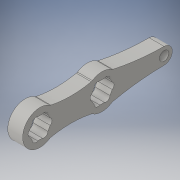
# Autodesk Inventor part: Kevin_CAD_test
Saved by Autodesk Inventor 2016 (Build 200138000, 138)
## iProperties
Created: 2018-06-19
Part Number: Kevin_CAD_test
Material: Generic
Document SubType Name: Modeling
Designer: Student
Density: 1 g/cm^3
Appearance: Default
Author: Student
Autodesk Inventor part; units mm, degrees
ref_plane "YZ Plane" through (0, 0, 0) normal (1, 0, 0) x (0, 1, 0)
ref_plane "XZ Plane" through (0, 0, 0) normal (0, 1, 0) x (-1, 0, 0)
ref_plane "XY Plane" through (0, 0, 0) normal (0, 0, 1) x (1, 0, 0)
sketch "Sketch1" plane through (0, 0, 0) normal (1, 0, 0) x (0, 1, 0)
  arc A0 (14.7437, -9.9374) -> (-14.7437, -9.9374) centre (0, 0) ccw
  arc A1 (-8.382, -127) -> (8.382, -127) centre (0, -127) ccw
  line L0 (-3.2996, -10.4245) -> (-7.3781, -8.0697)
  line L1 (-10.6776, -2.3547) -> (-10.6776, 2.3547)
  line L2 (-7.3781, 8.0697) -> (-3.2996, 10.4245)
  line L3 (3.2996, 10.4245) -> (7.3781, 8.0697)
  line L4 (10.6776, 2.3547) -> (10.6776, -2.3547)
  line L5 (7.3781, -8.0697) -> (3.2996, -10.4245)
  arc A2 (10.6776, 2.3547) -> (7.3781, 8.0697) centre (7.3781, 4.2597) ccw
  arc A3 (7.3781, -8.0697) -> (10.6776, -2.3547) centre (7.3781, -4.2597) ccw
  arc A4 (3.2996, 10.4245) -> (-3.2996, 10.4245) centre (0, 8.5195) ccw
  arc A5 (-7.3781, 8.0697) -> (-10.6776, 2.3547) centre (-7.3781, 4.2597) ccw
  arc A6 (-10.6776, -2.3547) -> (-7.3781, -8.0697) centre (-7.3781, -4.2597) ccw
  arc A7 (-3.2996, -10.4245) -> (3.2996, -10.4245) centre (0, -8.5195) ccw
  line L6 (-3.2996, -73.9245) -> (-7.3781, -71.5697)
  line L7 (-10.6776, -65.8547) -> (-10.6776, -61.1453)
  line L8 (-7.3781, -55.4303) -> (-3.2996, -53.0755)
  line L9 (3.2996, -53.0755) -> (7.3781, -55.4303)
  line L10 (10.6776, -61.1453) -> (10.6776, -65.8547)
  line L11 (7.3781, -71.5697) -> (3.2996, -73.9245)
  arc A8 (10.6776, -61.1453) -> (7.3781, -55.4303) centre (7.3781, -59.2403) ccw
  arc A9 (7.3781, -71.5697) -> (10.6776, -65.8547) centre (7.3781, -67.7597) ccw
  arc A10 (3.2996, -53.0755) -> (-3.2996, -53.0755) centre (0, -54.9805) ccw
  arc A11 (-7.3781, -55.4303) -> (-10.6776, -61.1453) centre (-7.3781, -59.2403) ccw
  arc A12 (-10.6776, -65.8547) -> (-7.3781, -71.5697) centre (-7.3781, -67.7597) ccw
  arc A13 (-3.2996, -73.9245) -> (3.2996, -73.9245) centre (0, -72.0195) ccw
  circle A14 centre (0, -127) radius 4.765
  arc A15 (14.268, -11.0656) -> (14.268, -52.4344) centre (113.7401, -31.75) ccw
  arc A16 (-14.268, -52.4344) -> (-14.268, -11.0656) centre (-113.7401, -31.75) ccw
  arc A17 (14.2667, -74.5446) -> (8.382, -127) centre (262.3746, -128.9362) ccw
  arc A18 (-8.382, -127) -> (-14.2667, -74.5446) centre (-262.3746, -128.9362) ccw
  arc A19 (14.7365, -73.4481) -> (14.7437, -53.5626) centre (0, -63.5) ccw
  arc A20 (-14.7437, -53.5626) -> (-14.7365, -73.4481) centre (0, -63.5) ccw
  arc A21 (14.7365, -73.4481) -> (14.2667, -74.5446) centre (17.368, -75.2245) ccw
  arc A22 (14.268, -52.4344) -> (14.7437, -53.5626) centre (17.3765, -51.788) ccw
  arc A23 (-14.7437, -53.5626) -> (-14.268, -52.4344) centre (-17.3765, -51.788) ccw
  arc A24 (-14.2667, -74.5446) -> (-14.7365, -73.4481) centre (-17.368, -75.2245) ccw
  arc A25 (-14.268, -11.0656) -> (-14.7437, -9.9374) centre (-17.3765, -11.712) ccw
  arc A26 (14.7437, -9.9374) -> (14.268, -11.0656) centre (17.3765, -11.712) ccw
  dimension "d0" = 35.56
  dimension "d21" = 16.764
  dimension "d34" = 9.5301
  dimension "d35" = 101.6
  dimension "d36" = 101.6
  dimension "d37" = 254
  dimension "d38" = 254
  dimension "d39" = 3.175
  constraints: 52 point on circle, 27 centre point, 24 end point, 12 tangent, 5 equal radius, 3 coincident, 14 other
  measures "d0" diameter of A0
  measures "d21" diameter of A1
  measures "d34" diameter of A14
  measures "d35" radius of A15
  measures "d36" radius of A16
  measures "d37" radius of A17
  measures "d38" radius of A18
  measures "d39" radius of A21
extrude "Extrusion1" add sketch "Sketch1" along normal blind 15.24
body "Solid1"
